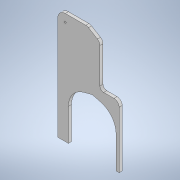
# Autodesk Inventor part: guarra
Saved by Autodesk Inventor 2020 (Build 240168000, 168)
## iProperties
Created: 2020-04-22
Part Number: guarra
Material: Genérico
Document SubType Name: Modeling
Designer: gi-se
Density: 1 g/cm^3
Appearance: Padrão
Author: gi-se
Autodesk Inventor part; units mm, degrees
ref_plane "YZ Plane" through (0, 0, 0) normal (1, 0, 0) x (0, 1, 0)
ref_plane "XZ Plane" through (0, 0, 0) normal (0, 1, 0) x (-1, 0, 0)
ref_plane "XY Plane" through (0, 0, 0) normal (0, 0, 1) x (1, 0, 0)
sketch "Esboço1" plane through (0, 0, 0) normal (0, 0, 1) x (1, 0, 0)
  circle A0 centre (0, 0) radius 0.8 projected
  circle A1 centre (37.4, -29.1) radius 15.2 projected
  line L0 (50.6, -101.1) -> (52.6, -101.1)
  line L1 (52.6, -101.1) -> (52.6, -45.7)
  line L2 (5.4, 7.4) -> (20.0215, 7.4)
  arc A2 (0, 7.4) -> (-7.2767, -1.3455) centre (0, 0) ccw
  line L3 (33.8, -29.1) -> (33.8, -2.8388)
  line L4 (31.3623, 1.4548) -> (22.5838, 6.6936)
  arc A3 (33.8, -37.1) -> (41, -37.1) centre (37.4, -37.1) ccw projected
  line L5 (33.8, -37.1) -> (33.8, -29.1)
  line L6 (37.4, -40.7) -> (47.6, -40.7)
  line L7 (0, 7.4) -> (7.6354, 7.4)
  line L8 (27.5941, -48.4938) -> (34.7764, -50.4183)
  line L9 (52.6, -101.1) -> (49.6, -101.1)
  line L10 (49.6, -101.1) -> (49.6, -69.7368)
  line L11 (52.6, -54.3903) -> (52.6, -101.1)
  arc A4 (49.6, -69.7368) -> (34.7764, -50.4183) centre (29.6, -69.7368) ccw
  arc A5 (52.6, -45.7) -> (47.6, -40.7) centre (47.6, -45.7) ccw
  arc A6 (22.5838, 6.6936) -> (20.0215, 7.4) centre (20.0215, 2.4) ccw
  arc A7 (33.8, -2.8388) -> (31.3623, 1.4548) centre (28.8, -2.8388) ccw
  line L12 (2, -101.1) -> (0, -101.1)
  line L13 (52.6, -51.1) -> (1.2194, -51.1) construction
  line L14 (25.0059, -48.4938) -> (17.8236, -50.4183)
  line L15 (0, -101.1) -> (3, -101.1)
  line L16 (3, -101.1) -> (3, -69.7368)
  arc A8 (17.8236, -50.4183) -> (3, -69.7368) centre (23, -69.7368) ccw
  circle A9 centre (0, 0) radius 7.4
  arc A10 (27.5941, -48.4938) -> (25.0059, -48.4938) centre (26.3, -53.3234) ccw
  line L17 (-7.4, 0) -> (-7.4, -101.1)
  line L18 (-7.4, -101.1) -> (0, -101.1)
  point P0 (21.4, 7.4)
  point P1 (49.6, -54.3903)
  point P2 (3, -54.3903)
  point P3 (49.5452, -41.9185)
  dimension "d7" = 20
  dimension "d9" = 5
  dimension "d11" = 5
  constraints: 38 end point, 15 point on circle, 12 tangent, 7 centre point, 7 point on line, 3 vertical, 2 coincident, 1 collinear, 1 equal radius, 1 horizontal, 1 horizontal alignment, 1 parallel, 1 perpendicular, 3 other
  measures "d7" radius of A4
  measures "d9" radius of A6
  measures "d11" radius of A10
extrude "Extrusão1" add sketch "Esboço1" against normal blind 3 contours L3 L5 A3 L6 A1 | A1 L6 A5 L1 L0 L9 L10 A4 L8 A10 L14 A8 L16 L15 L12 L18 L17 A2 A9 L7 L2 A6 L4 A7 L3 | A9 A2 picked at (30.2417, -33.5073)
